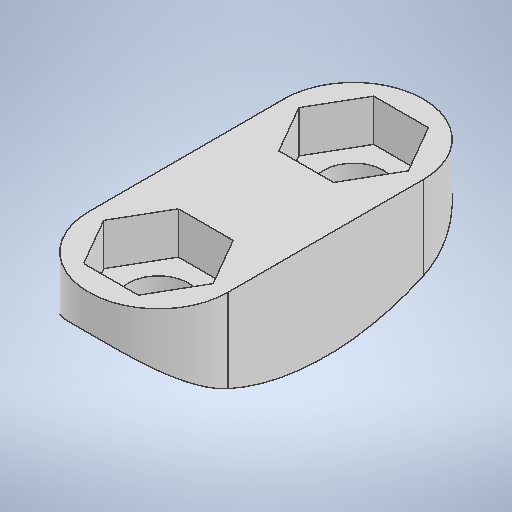
# Autodesk Inventor part: Spacer_Collective_Base_NutM4
Saved by Autodesk Inventor 2026.2 (Build 302298000, 298)
## iProperties
Created: 2026-03-24
Part Number: Spacer_Collective_Base_NutM4
Material: Generic
Document SubType Name: Modeling
Designer: Paco Ariel
Density: 1 g/cm^3
Appearance: Default
Author: Paco Ariel
Autodesk Inventor part; units mm, degrees
ref_plane "YZ Plane" through (0, 0, 0) normal (1, 0, 0) x (0, 1, 0)
ref_plane "XZ Plane" through (0, 0, 0) normal (0, 1, 0) x (-1, 0, 0)
ref_plane "XY Plane" through (0, 0, 0) normal (0, 0, 1) x (1, 0, 0)
sketch "Sketch1" plane through (0, 0, 0) normal (0, 1, 0) x (-1, 0, 0)
  arc A0 (-5, 0) -> (5, 0) centre (0, 0) ccw
  circle A1 centre (0, 0) radius 2.15
  arc A2 (5, 14) -> (-5, 14) centre (0, 14) ccw
  circle A3 centre (0, 14) radius 2.15
  line L0 (-5, 0) -> (-5, 14)
  line L1 (5, 0) -> (5, 14)
  line L2 (0, 0) -> (0, 2.15)
  line L3 (0, 9) -> (0, 14)
  dimension "d1" = 4.3
  dimension "d0" = 10
  dimension "d9" = 14
  dimension "d10" = 10
  dimension "d11" = 4.3
  constraints: 8 end point, 4 coincident, 4 point on circle, 3 centre point, 3 vertical, 2 tangent, 1 parallel, 1 vertical alignment, 2 other
  measures "d0" diameter of A0
  measures "d9" distance of L2.start L3.end
  measures "d10" diameter of A2
  measures "d11" diameter of A3
extrude "Extrusion1" add sketch "Sketch1" along normal blind 10
sketch "Sketch2" plane through (0, 10, 0) normal (0, 1, 0) x (-1, 0, 0)
  line L0 (1.963, 3.4) -> (3.926, 0)
  line L1 (3.926, 0) -> (1.963, -3.4)
  line L2 (1.963, -3.4) -> (-1.963, -3.4)
  line L3 (-1.963, -3.4) -> (-3.926, 0)
  line L4 (-3.926, 0) -> (-1.963, 3.4)
  line L5 (-1.963, 3.4) -> (1.963, 3.4)
  circle A0 centre (0, 14) radius 2.15 projected
  line L6 (-3.926, 14) -> (-1.963, 17.4)
  line L7 (-1.963, 17.4) -> (1.963, 17.4)
  line L8 (1.963, 17.4) -> (3.926, 14)
  line L9 (3.926, 14) -> (1.963, 10.6)
  line L10 (1.963, 10.6) -> (-1.963, 10.6)
  line L11 (-1.963, 10.6) -> (-3.926, 14)
  point P0 (0, 0)
  point P1 (0, 0)
  dimension "d4" = 6.8
  constraints: 24 end point, 2 coincident, 26 other
  measures "d4" distance between parallel lines of L5 L2
extrude "Extrusion2" cut sketch "Sketch2" against normal blind 3
sketch "Sketch3" plane through (0, 0, 0) normal (1, 0, 0) x (0, 1, 0)
  line L0 (0, 0) -> (0, 7)
  line L1 (0, 2.15) -> (0, -2.15) projected
  line L2 (0, 7) -> (19.5, 7)
  circle A0 centre (19.5, 7) radius 17
  line L3 (7, -2.15) -> (7, 2.15) projected
  line L4 (7, 0) -> (7, 3.4) projected
  line L5 (7, -3.4) -> (7, 0) projected
  line L6 (7, 0) -> (7, -3.4) projected
  line L7 (7, 3.4) -> (7, 0) projected
  circle A1 centre (19.5, 7) radius 30.634
  dimension "d7" = 7
  dimension "d8" = 19.5
  dimension "d12" = 34
  constraints: 4 end point, 2 centre point, 2 coincident, 1 collinear, 1 perpendicular
  measures "d7" distance of L0.start L0.end
  measures "d8" distance of L0.end L2.end
  measures "d12" diameter of A0
extrude "Extrusion3" cut sketch "Sketch3" along normal through all both and the other way through all
body "Solid1"
